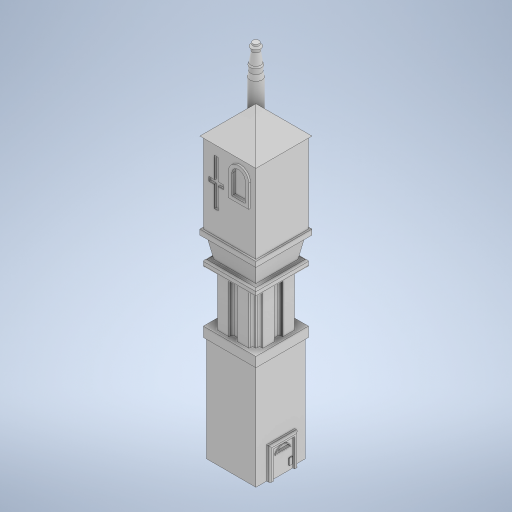
# Autodesk Inventor part: 背部建築
Saved by Autodesk Inventor 2024 (Build 280153000, 153)
## iProperties
Created: 2024-05-24
Part Number: 背部建築
Material: 一般
Document SubType Name: Modeling
Designer: User
Density: 1 g/cm^3
Appearance: 預設
Author: User
Autodesk Inventor part; units mm, degrees
ref_plane "YZ Plane" through (0, 0, 0) normal (1, 0, 0) x (0, 1, 0)
ref_plane "XZ Plane" through (0, 0, 0) normal (0, 1, 0) x (-1, 0, 0)
ref_plane "XY Plane" through (0, 0, 0) normal (0, 0, 1) x (1, 0, 0)
sketch "草圖1" plane through (0, 0, 0) normal (0, 1, 0) x (-1, 0, 0)
  line L0 (-7.5, 7.5) -> (7.5, 7.5)
  line L1 (7.5, 7.5) -> (7.5, -7.5)
  line L2 (7.5, -7.5) -> (-7.5, -7.5)
  line L3 (-7.5, -7.5) -> (-7.5, 7.5)
  line L4 (-7.5, 7.5) -> (7.5, -7.5) construction
  line L5 (7.5, 7.5) -> (-7.5, -7.5) construction
  point P0 (0, 0)
  dimension "d0" = 15
  dimension "d1" = 15
  constraints: 12 end point, 2 midpoint, 2 parallel, 1 horizontal, 1 perpendicular
  measures "d0" distance of L1.end L2.end
  measures "d1" distance of L0.end L1.end
extrude "擠出1" add sketch "草圖1" along normal blind 2.8
sketch "草圖2" plane through (0, 2.8, 0) normal (0, 1, 0) x (1, 0, 0)
  line L0 (5.5, -5.5) -> (-5.5, -5.5)
  line L1 (-5.5, -5.5) -> (-5.5, 5.5)
  line L2 (-5.5, 5.5) -> (5.5, 5.5)
  line L3 (5.5, 5.5) -> (5.5, -5.5)
  line L4 (5.5, -5.5) -> (-5.5, 5.5) construction
  line L5 (-5.5, -5.5) -> (5.5, 5.5) construction
  point P0 (0, 0)
  dimension "d4" = 11
  dimension "d5" = 11
  constraints: 12 end point, 2 midpoint, 2 parallel, 1 horizontal, 1 perpendicular
  measures "d4" distance of L1.end L2.end
  measures "d5" distance of L0.end L1.end
extrude "擠出2" add sketch "草圖2" along normal blind 14.5
sketch "草圖4" plane through (0, 17.3, 0) normal (0, 1, 0) x (1, 0, 0)
  line L0 (-5.5, -5.5) -> (-5.5, 5.5) projected
  line L1 (-5.5, -4.5) -> (-6.5, -4.5)
  line L2 (-6.5, -4.5) -> (-6.5, -1.2)
  line L3 (-6.5, -1.2) -> (-5.5, -1.2)
  line L4 (-5.5, -1.2) -> (-5.5, -4.5)
  line L5 (-5.5, 1.2) -> (-6.5, 1.2)
  line L6 (-6.5, 1.2) -> (-6.5, 4.5)
  line L7 (-6.5, 4.5) -> (-5.5, 4.5)
  line L8 (-5.5, 4.5) -> (-5.5, 1.2)
  line L9 (5.5, 5.5) -> (-5.5, 5.5) projected
  line L10 (-5.5, -5.5) -> (5.5, -5.5) projected
  line L11 (-4.5, 5.5) -> (-1.2, 5.5)
  line L12 (-1.2, 5.5) -> (-1.2, 6.5)
  line L13 (-1.2, 6.5) -> (-4.5, 6.5)
  line L14 (-4.5, 6.5) -> (-4.5, 5.5)
  line L15 (1.2, 5.5) -> (4.5, 5.5)
  line L16 (4.5, 5.5) -> (4.5, 6.5)
  line L17 (4.5, 6.5) -> (1.2, 6.5)
  line L18 (1.2, 6.5) -> (1.2, 5.5)
  line L19 (5.5, 5.5) -> (5.5, -5.5) projected
  line L20 (5.5, -1.2) -> (6.5, -1.2)
  line L21 (6.5, -1.2) -> (6.5, -4.5)
  line L22 (6.5, -4.5) -> (5.5, -4.5)
  line L23 (5.5, -4.5) -> (5.5, -1.2)
  line L24 (5.5, 1.2) -> (6.5, 1.2)
  line L25 (6.5, 1.2) -> (6.5, 4.5)
  line L26 (6.5, 4.5) -> (5.5, 4.5)
  line L27 (5.5, 4.5) -> (5.5, 1.2)
  line L28 (-4.5, -5.5) -> (-1.2, -5.5)
  line L29 (-1.2, -5.5) -> (-1.2, -6.5)
  line L30 (-1.2, -6.5) -> (-4.5, -6.5)
  line L31 (-4.5, -6.5) -> (-4.5, -5.5)
  line L32 (5.5, -5.5) -> (-5.5, -5.5) projected
  line L33 (1.2, -5.5) -> (4.5, -5.5)
  line L34 (4.5, -5.5) -> (4.5, -6.5)
  line L35 (4.5, -6.5) -> (1.2, -6.5)
  line L36 (1.2, -6.5) -> (1.2, -5.5)
  point P0 (0, 0)
  dimension "d8" = 1
  dimension "d9" = 3.3
  dimension "d10" = 1
  dimension "d11" = 3.3
  dimension "d12" = 1
  dimension "d13" = 1
  dimension "d14" = 3.3
  dimension "d15" = 1
  dimension "d16" = 3.3
  dimension "d17" = 1
  dimension "d20" = 1
  dimension "d21" = 1
  dimension "d22" = 3.3
  dimension "d23" = 1
  constraints: 64 end point, 16 parallel, 9 point on line, 8 horizontal, 8 perpendicular
  measures "d8" distance of L2.end L3.end
  measures "d9" distance of L1.end L2.end
  measures "d10" distance of L6.end L7.end
  measures "d11" distance of L5.end L6.end
  measures "d12" distance between parallel lines of L9 L7
  measures "d13" distance between parallel lines of L10 L1
  measures "d14" distance of L13.end L12.end
  measures "d15" distance of L12.end L11.end
  measures "d16" distance of L17.end L16.end
  measures "d17" distance of L16.end L15.end
  measures "d20" distance between parallel lines of L19 L16
  measures "d21" distance between parallel lines of L0 L14
  measures "d22" distance of L29.end L30.end
  measures "d23" distance of L28.end L29.end
extrude "擠出3" add sketch "草圖4" against normal blind 14.5 contours L1 L2 L3 L0 | L10 L29 L30 L31 | L5 L6 L7 L0 | L10 L34 L35 L36 | L14 L13 L12 L9 | L19 L20 L21 L22 | L18 L17 L16 L9 | L19 L26 L25 L24
sketch "草圖5" plane through (0, 17.3, 0) normal (0, 1, 0) x (1, 0, 0)
  line L0 (-7.5, -7.5) -> (7.5, -7.5) projected
  line L1 (7.5, -7.5) -> (7.5, 7.5) projected
  line L2 (-7.5, -7.5) -> (7.5, -7.5)
  line L3 (7.5, -7.5) -> (7.5, 7.5)
  line L4 (7.5, 7.5) -> (-7.5, 7.5)
  line L5 (-7.5, 7.5) -> (-7.5, -7.5)
  point P0 (0, 0)
  constraints: 8 end point, 2 parallel, 1 horizontal, 1 perpendicular
extrude "擠出4" add sketch "草圖5" along normal blind 2
sketch "草圖6" plane through (0, 19.3, 0) normal (0, 1, 0) x (1, 0, 0)
  line L0 (6, -6) -> (-6, -6)
  line L1 (-6, -6) -> (-6, 6)
  line L2 (-6, 6) -> (6, 6)
  line L3 (6, 6) -> (6, -6)
  line L4 (6, -6) -> (-6, 6) construction
  line L5 (-6, -6) -> (6, 6) construction
  point P0 (0, 0)
  dimension "d28" = 12
  dimension "d29" = 12
  constraints: 12 end point, 2 midpoint, 2 parallel, 1 horizontal, 1 perpendicular
  measures "d28" distance of L1.end L2.end
  measures "d29" distance of L0.end L1.end
extrude "擠出5" add sketch "草圖6" along normal blind 6 draft 10
sketch "草圖7" plane through (0, 25.3, 0) normal (0, 1, 0) x (1, 0, 0)
  line L0 (-7.5, 7.5) -> (-7.5, -7.5) projected
  line L1 (7.5, -7.5) -> (-7.5, -7.5)
  line L2 (-7.5, -7.5) -> (-7.5, 7.5)
  line L3 (-7.5, 7.5) -> (7.5, 7.5)
  line L4 (7.5, 7.5) -> (7.5, -7.5)
  line L5 (7.5, -7.5) -> (-7.5, 7.5) construction
  line L6 (-7.5, -7.5) -> (7.5, 7.5) construction
  line L7 (8, -8) -> (-8, -8)
  line L8 (-8, -8) -> (-8, 8)
  line L9 (-8, 8) -> (8, 8)
  line L10 (8, 8) -> (8, -8)
  line L11 (8, -8) -> (-8, 8) construction
  line L12 (-8, -8) -> (8, 8) construction
  point P0 (0, 0)
  dimension "d32" = 16
  dimension "d33" = 16
  constraints: 24 end point, 4 midpoint, 4 parallel, 2 horizontal, 2 perpendicular
  measures "d32" distance of L8.end L9.end
  measures "d33" distance of L7.end L8.end
extrude "擠出6" add sketch "草圖7" along normal blind 1.5 contours L3 L4 L1 L0 | L7 L8 L9 L10
fillet "圓角1" radius 0.5 24 edges at (7.5, 19.3, 0) (7.5, 17.3, 0) (0, 19.3, -7.5) (0, 17.3, -7.5) (-7.5, 19.3, 0) (-7.5, 17.3, 0) (0, 19.3, 7.5) (0, 17.3, 7.5) (1.2, 10.05, -5.5) (-1.2, 10.05, -5.5) (-4.5, 10.05, -5.5) (-5.5, 10.05, -4.5) (-5.5, 10.05, -1.2) (-5.5, 10.05, 1.2) (-5.5, 10.05, 4.5) (-4.5, 10.05, 5.5) (-1.2, 10.05, 5.5) (1.2, 10.05, 5.5) (4.5, 10.05, 5.5) (5.5, 10.05, 4.5) (5.5, 10.05, 1.2) (5.5, 10.05, -1.2) (5.5, 10.05, -4.5) (4.5, 10.05, -5.5)
sketch "草圖8" plane through (0, 26.8, 0) normal (0, 1, 0) x (1, 0, 0)
  line L0 (-7.5, 7.5) -> (-7.5, -7.5) projected
  line L1 (7.5, -7.5) -> (-7.5, -7.5)
  line L2 (-7.5, -7.5) -> (-7.5, 7.5)
  line L3 (-7.5, 7.5) -> (7.5, 7.5)
  line L4 (7.5, 7.5) -> (7.5, -7.5)
  line L5 (7.5, -7.5) -> (-7.5, 7.5) construction
  line L6 (-7.5, -7.5) -> (7.5, 7.5) construction
  point P0 (0, 0)
  constraints: 12 end point, 2 midpoint, 2 parallel, 1 horizontal, 1 perpendicular
extrude "擠出7" add sketch "草圖8" along normal blind 23
sketch "草圖9" plane through (0, 49.8, 0) normal (0, 1, 0) x (1, 0, 0)
  line L0 (-8, 8) -> (-8, -8) projected
  line L1 (8, -8) -> (-8, -8)
  line L2 (-8, -8) -> (-8, 8)
  line L3 (-8, 8) -> (8, 8)
  line L4 (8, 8) -> (8, -8)
  line L5 (8, -8) -> (-8, 8) construction
  line L6 (-8, -8) -> (8, 8) construction
  point P0 (0, 0)
  constraints: 12 end point, 2 midpoint, 2 parallel, 1 horizontal, 1 perpendicular
extrude "擠出8" add sketch "草圖9" along normal blind 10 draft -45
sketch "草圖10" plane through (0, 26.8, 0) normal (0, 1, 0) x (1, 0, 0)
  line L0 (-8, 8) -> (0, 0) projected
  circle A0 centre (-2.7531, 2.7531) radius 1.75
  dimension "d41" = 3.5
  constraints: 1 centre point, 1 point on line
  measures "d41" diameter of A0
extrude "擠出9" add sketch "草圖10" along normal blind 35
sketch "草圖11" plane through (-2.7531, 61.8, -2.7531) normal (0, 1, 0) x (1, 0, 0)
  circle A0 centre (0, 0) radius 1.75
  point P0 (2.7531, -2.7531)
  constraints: 1 centre point
extrude "擠出10" add sketch "草圖11" along normal blind 1.5 draft -10
sketch "草圖12" plane through (-2.7531, 63.3, -2.7531) normal (0, 1, 0) x (1, 0, 0)
  circle A0 centre (0, 0) radius 1.4855 projected
  circle A1 centre (0, 0) radius 1.4855
  point P0 (2.7531, -2.7531)
  constraints: 1 centre point, 1 coincident
extrude "擠出11" add sketch "草圖12" along normal blind 1.5 draft 5
sketch "草圖13" plane through (-2.7531, 64.8, -2.7531) normal (0, 1, 0) x (1, 0, 0)
  circle A0 centre (0, 0) radius 1.6167
  point P0 (2.7531, -2.7531)
  constraints: 1 centre point, 1 coincident
extrude "擠出12" add sketch "草圖13" along normal blind 0.5 draft -20
sketch "草圖14" plane through (-2.7531, 65.3, -2.7531) normal (0, 1, 0) x (1, 0, 0)
  circle A0 centre (0, 0) radius 1.4348
  point P0 (2.7531, -2.7531)
  constraints: 1 centre point
extrude "擠出13" add sketch "草圖14" along normal blind 3 draft -8
sketch "草圖15" plane through (-2.7531, 68.3, -2.7531) normal (0, 1, 0) x (1, 0, 0)
  circle A0 centre (0, 0) radius 1.6167 projected
  circle A1 centre (0, 0) radius 1.0131
  point P0 (2.7531, -2.7531)
  constraints: 1 centre point, 1 coincident
extrude "擠出14" add sketch "草圖15" along normal blind 1 draft 20 contours A1
sketch "草圖16" plane through (-2.7531, 69.3, -2.7531) normal (0, 1, 0) x (1, 0, 0)
  circle A0 centre (0, 0) radius 1.3771
  point P0 (2.7531, -2.7531)
  constraints: 1 centre point
extrude "擠出15" add sketch "草圖16" along normal blind 0.5 draft -45
sketch "草圖18" plane through (-2.7531, 69.8, -2.7531) normal (0, 1, 0) x (1, 0, 0)
  circle A0 centre (0, 0) radius 0.8771
  point P0 (2.7531, -2.7531)
  constraints: 1 centre point
extrude "擠出17" add sketch "草圖18" along normal blind 0.5
sketch "草圖19" plane through (7.5, 26.8, -7.5) normal (0, 0, -1) x (-1, 0, 0)
  line L0 (6.3618, 12.8306) -> (2.5618, 12.8306)
  line L1 (2.5618, 12.8306) -> (2.5618, 18.3306)
  line L2 (2.5618, 18.3306) -> (6.3618, 18.3306)
  line L3 (6.3618, 18.3306) -> (6.3618, 12.8306)
  line L4 (6.3618, 12.8306) -> (2.5618, 18.3306) construction
  line L5 (2.5618, 12.8306) -> (6.3618, 18.3306) construction
  arc A0 (6.3618, 18.3306) -> (2.5618, 18.3306) centre (4.4618, 18.3306) ccw
  arc A1 (7.3618, 18.3306) -> (1.5618, 18.3306) centre (4.4618, 18.3306) ccw
  line L6 (7.3618, 18.3306) -> (7.3618, 11.8306)
  line L7 (7.3618, 11.8306) -> (1.5618, 11.8306)
  line L8 (1.5618, 11.8306) -> (1.5618, 18.3306)
  point P0 (7.5, -26.8)
  point P1 (4.4618, 15.5806)
  dimension "d60" = 3.8
  dimension "d61" = 5.5
  dimension "d62" = 1
  dimension "d63" = 1
  constraints: 18 end point, 4 point on circle, 3 parallel, 2 centre point, 2 midpoint, 2 perpendicular, 2 tangent, 1 horizontal, 2 other
  measures "d60" distance of L1.end L2.end
  measures "d61" distance of L0.end L1.end
  measures "d62" radial gap between concentric circles of A0 A1
  measures "d63" distance between parallel lines of L3 L6
extrude "擠出18" add sketch "草圖19" along normal blind 0.5
extrude "擠出19" cut sketch "草圖19" against normal blind 0.5 contours L0 L1 L2 L3 | L2 A0
sketch "草圖20" plane through (7.5, 26.8, -7.5) normal (0, 0, -1) x (-1, 0, 0)
  line L0 (9.3399, 12.7015) -> (13.3399, 12.7015)
  line L1 (13.3399, 12.7015) -> (13.3399, 13.7015)
  line L2 (13.3399, 13.7015) -> (9.3399, 13.7015)
  line L3 (9.3399, 13.7015) -> (9.3399, 12.7015)
  line L4 (9.3399, 12.7015) -> (13.3399, 13.7015) construction
  line L5 (13.3399, 12.7015) -> (9.3399, 13.7015) construction
  line L6 (10.8399, 6.7015) -> (11.8399, 6.7015)
  line L7 (11.8399, 6.7015) -> (11.8399, 19.7015)
  line L8 (11.8399, 19.7015) -> (10.8399, 19.7015)
  line L9 (10.8399, 19.7015) -> (10.8399, 6.7015)
  line L10 (10.8399, 6.7015) -> (11.8399, 19.7015) construction
  line L11 (11.8399, 6.7015) -> (10.8399, 19.7015) construction
  point P0 (7.5, -26.8)
  point P1 (11.3399, 13.2015)
  point P2 (11.3399, 13.2015)
  point P3 (10.8399, 13.7015)
  point P4 (10.8399, 12.7015)
  point P5 (11.8399, 12.7015)
  point P6 (11.8399, 13.7015)
  dimension "d68" = 4
  dimension "d69" = 1
  dimension "d70" = 13
  dimension "d71" = 1
  constraints: 24 end point, 5 midpoint, 4 parallel, 2 horizontal, 2 perpendicular
  measures "d68" distance of L2.end L1.end
  measures "d69" distance of L8.end L7.end
  measures "d70" distance of L7.end L6.end
  measures "d71" distance of L0.end L1.end
extrude "擠出20" cut sketch "草圖20" against normal blind 0.5
fillet "圓角2" radius 0.1 12 edges at (-3.3399, 43.5015, -7.5) (-4.3399, 43.5015, -7.5) (-5.0899, 40.5015, -7.5) (-5.8399, 40.0015, -7.5) (-3.8399, 46.5015, -7.5) (-1.8399, 40.0015, -7.5) (-2.5899, 40.5015, -7.5) (-2.5899, 39.5015, -7.5) (-3.3399, 36.5015, -7.5) (-4.3399, 36.5015, -7.5) (-5.0899, 39.5015, -7.5) (-3.8399, 33.5015, -7.5)
fillet "圓角3" radius 0.5 8 edges at (5.9382, 41.8806, -8) (0.1382, 41.8806, -8) (3.0382, 48.0306, -8) (1.1382, 42.3806, -8) (4.9382, 42.3806, -8) (3.0382, 47.0306, -8) (3.0382, 39.6306, -8) (3.0382, 38.6306, -8)
sketch "草圖21" plane through (-7.5, 26.8, -7.5) normal (-1, 0, 0) x (0, 0, 1)
  line L0 (4.5, 2.4438) -> (10.5, 2.4438)
  line L1 (10.5, 2.4438) -> (10.5, 10.4438)
  line L2 (10.5, 10.4438) -> (4.5, 10.4438)
  line L3 (4.5, 10.4438) -> (4.5, 2.4438)
  line L4 (4.5, 2.4438) -> (10.5, 10.4438) construction
  line L5 (10.5, 2.4438) -> (4.5, 10.4438) construction
  arc A0 (10.5, 10.4438) -> (4.5, 10.4438) centre (7.5, 10.4438) ccw
  point P0 (7.5, -26.8)
  point P1 (7.5, 6.4438)
  dimension "d76" = 6
  dimension "d77" = 8
  constraints: 12 end point, 2 midpoint, 2 parallel, 2 point on circle, 2 tangent, 1 centre point, 1 horizontal, 1 perpendicular
  measures "d76" distance of L2.end L1.end
  measures "d77" distance of L1.end L0.end
extrude "擠出21" cut sketch "草圖21" against normal blind 0.5
mirror "鏡射1" about plane through (0, 0, 0) normal (0, 0, 1) of "擠出19", "擠出18", "擠出20", "圓角2"
sketch "草圖22" plane through (0, 0, 0) normal (0, -1, 0) x (1, 0, 0)
  line L0 (6, -6) -> (7.058, -7.058) projected
  line L1 (-7.058, 7.058) -> (7.058, 7.058)
  line L2 (7.058, 7.058) -> (7.058, -7.058)
  line L3 (7.058, -7.058) -> (-7.058, -7.058)
  line L4 (-7.058, -7.058) -> (-7.058, 7.058)
  line L5 (-8, 8) -> (0, 0) projected
  line L6 (-7.058, 7.058) -> (7.058, -7.058) construction
  line L7 (7.058, 7.058) -> (-7.058, -7.058) construction
  constraints: 12 end point, 2 midpoint, 2 parallel, 1 horizontal, 1 perpendicular
extrude "擠出22" add sketch "草圖22" along normal blind 30
sketch "草圖23" plane through (7.058, 0, 7.058) normal (1, 0, 0) x (0, 0, -1)
  line L0 (14.1159, -30) -> (0, -30) projected
  line L1 (3.0579, -30) -> (11.0579, -30)
  line L2 (11.0579, -30) -> (11.0579, -21)
  line L3 (11.0579, -21) -> (3.0579, -21)
  line L4 (3.0579, -21) -> (3.0579, -30)
  line L5 (14.1159, 0) -> (14.1159, -30) projected
  line L6 (0, 0) -> (0, -30) projected
  line L7 (4.0579, -30) -> (10.0579, -30)
  line L8 (10.0579, -30) -> (10.0579, -22)
  line L9 (10.0579, -22) -> (4.0579, -22)
  line L10 (4.0579, -22) -> (4.0579, -30)
  line L11 (7.0579, -23.9653) -> (9.0579, -23.9653)
  line L12 (7.0579, -23.9653) -> (5.0579, -23.9653)
  arc A0 (9.0579, -23.9653) -> (5.0579, -23.9653) centre (7.0579, -24.8818) ccw
  line L13 (9.3485, -24.1653) -> (7.0579, -24.1653)
  line L14 (7.0579, -24.1653) -> (4.7674, -24.1653)
  arc A1 (9.3485, -24.1653) -> (4.7674, -24.1653) centre (7.0579, -24.8818) ccw
  point P0 (7.058, 0)
  dimension "d82" = 8
  dimension "d83" = 9
  dimension "d84" = 3.058
  dimension "d85" = 3.0579
  dimension "d86" = 1
  dimension "d87" = 1
  dimension "d88" = 1
  dimension "d89" = 2
  dimension "d90" = 2
  dimension "d91" = 2.2
  dimension "d96" = 0.2
  constraints: 24 end point, 4 horizontal, 4 parallel, 4 point on circle, 2 centre point, 2 perpendicular, 2 point on line, 2 other
  measures "d82" distance of L3.end L2.end
  measures "d83" distance of L2.end L1.end
  measures "d84" distance between parallel lines of L5 L2
  measures "d85" distance between parallel lines of L6 L4
  measures "d86" distance between parallel lines of L3 L9
  measures "d87" distance between parallel lines of L2 L8
  measures "d88" distance between parallel lines of L4 L10
  measures "d89" distance of L11.start L11.end
  measures "d90" distance of L11.start L12.end
  measures "d91" radius of A0
  measures "d96" distance between parallel lines of L11 L13
extrude "擠出23" add sketch "草圖23" along normal blind 1 contours L0 L8 L9 L10 L4 L3 L2
extrude "擠出24" add sketch "草圖23" along normal blind 0.5 contours L0 L10 L9 L8 | L13 L14 A1
extrude "擠出25" add sketch "草圖23" along normal blind 0.8 contours L13 L14 A1
sketch "草圖24" plane through (7.558, 0, 7.058) normal (1, 0, 0) x (0, 0, -1)
  line L0 (8.8504, -26.8366) -> (9.8504, -26.8366)
  line L1 (9.8504, -26.8366) -> (9.8504, -28.8366)
  line L2 (9.8504, -28.8366) -> (8.8504, -28.8366)
  line L3 (8.8504, -28.8366) -> (8.8504, -26.8366)
  point P0 (7.058, 0)
  dimension "d99" = 1
  dimension "d100" = 2
  constraints: 8 end point, 2 parallel, 1 horizontal, 1 perpendicular
  measures "d99" distance of L1.end L2.end
  measures "d100" distance of L0.end L1.end
extrude "擠出26" add sketch "草圖24" along normal blind 0.2
fillet "圓角4" radius 0.1 8 edges at (7.658, -26.8366, -1.7924) (7.758, -26.8366, -2.2924) (7.758, -27.8366, -1.7924) (7.758, -28.8366, -2.2924) (7.758, -27.8366, -2.7924) (7.658, -26.8366, -2.7924) (7.658, -28.8366, -2.7924) (7.658, -28.8366, -1.7924)
fillet "圓角5" radius 0.1 4 edges at (7.858, -22.4818, 0) (7.858, -22.6818, 0) (7.858, -23.9653, 0) (7.858, -24.1653, 0)
fillet "圓角6" radius 0.5 3 edges at (8.058, -21, 0) (8.058, -25.5, 4) (8.058, -25.5, -4)
